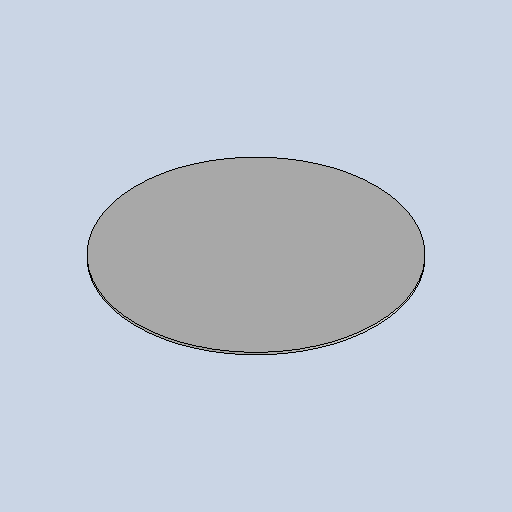
# Autodesk Inventor part: TKS 3111 top DS cup 1
Saved by Autodesk Inventor 2025.3 (Build 293356030, 356C)
## iProperties
Created: 2024-12-09
Part Number: TKS 3111 top DS cup 1
Material: Stainless Steel
Document SubType Name: Sheet Metal
Designer: admin
Mass: 3269.02 g
Surface Area: 1007.63 cm^2
Volume: 408.627 cm^3
Density: 8 g/cm^3
Flat Pattern Width: 21.5 cm
Flat Pattern Length: 21.5 cm
Flat Pattern Area: 462.25 cm^2
Sheet Metal Rule: AISI304 3mm Die 32
Sheet Metal Width: 215,000 mm
Sheet Metal Length: 215,000 mm
Sheet Metal Area: 46225,000 mm^2
Appearance: Default
Author: user
Autodesk Inventor part; units mm, degrees
ref_plane "YZ Plane" through (0, 0, 0) normal (1, 0, 0) x (0, 1, 0)
ref_plane "XZ Plane" through (0, 0, 0) normal (0, 1, 0) x (-1, 0, 0)
ref_plane "XY Plane" through (0, 0, 0) normal (0, 0, 1) x (1, 0, 0)
sketch "Sketch1" plane through (0, 0, 0) normal (0, 0, 1) x (1, 0, 0)
  circle A0 centre (0, 0) radius 107.5
  dimension "d22" = 215
  measures "d22" diameter of A0
extrude "Plate1" add sketch "Sketch1" along normal blind 2
equation "\"d2\" = Thickness"
equation "\"BendReliefWidth\" = Thickness"
equation "\"BendReliefDepth\" = 0.5 * Thickness"
equation "\"CornerReliefSize\" = 4 * Thickness"
equation "\"MinimumRemnant\" = 2 * Thickness"
equation "\"TransitionRadius\" = BendRadius"
equation "\"JacobiRadiusSize\" = BendRadius"
equation "\"GapSize\" = Thickness"
equation "\"Thickness\" = 2"
equation "\"BendRadius\" = 5"
body "Solid1"
